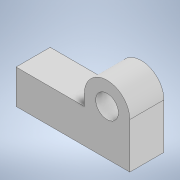
# Autodesk Inventor part: Peça1
Saved by Autodesk Inventor 2021 (Build 250183000, 183)
## iProperties
Created: 2022-02-01
Part Number: Peça1
Material: Genérico
Document SubType Name: Modeling
Designer: aluno
Density: 1 g/cm^3
Appearance: Padrão
Author: aluno
Autodesk Inventor part; units mm, degrees
ref_plane "YZ Plane" through (0, 0, 0) normal (1, 0, 0) x (0, 1, 0)
ref_plane "XZ Plane" through (0, 0, 0) normal (0, 1, 0) x (-1, 0, 0)
ref_plane "XY Plane" through (0, 0, 0) normal (0, 0, 1) x (1, 0, 0)
sketch "Esboço1" plane through (0, 0, 0) normal (0, 0, 1) x (1, 0, 0)
  line L0 (0, 0) -> (100, 0)
  line L1 (100, 0) -> (100, 40)
  line L2 (60, 40) -> (60, 30)
  line L3 (60, 30) -> (0, 30)
  line L4 (0, 30) -> (0, 0)
  arc A0 (100, 40) -> (60, 40) centre (80, 40) ccw
  dimension "d0" = 100
  dimension "d3" = 40
  dimension "d4" = 30
  dimension "d5" = 20
  constraints: 10 end point, 3 perpendicular, 2 horizontal, 2 point on circle, 2 tangent, 1 centre point, 1 coincident
  measures "d0" distance of L0.start L0.end
  measures "d3" distance of L0.end L1.end
  measures "d4" distance of L3.end L0.start
  measures "d5" radius of A0
extrude "Extrusão1" add sketch "Esboço1" along normal blind 30
sketch "Esboço2" plane through (0, 0, 30) normal (0, 0, 1) x (1, 0, 0)
  arc A0 (100, 40) -> (60, 40) centre (80, 40) ccw projected
  point P0 (0, 0)
  constraints: 1 coincident
hole "Furo1" at (80, 40, 30) direction (0, 0, -1) diameter 20 end through all
